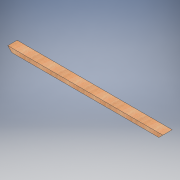
# Autodesk Inventor part: 58 Inch 45 Diagonal Piece
Saved by Autodesk Inventor 2016 (Build 200138000, 138)
## iProperties
Created: 2015-07-05
Part Number: 58 Inch 45 Diagonal Piece
Material: Wood (Birch)
Document SubType Name: Modeling
Designer: steele
Density: 0.55 g/cm^3
Appearance: Birch - Natural Polished
Author: steele
Autodesk Inventor part; units mm, degrees
ref_plane "YZ Plane" through (0, 0, 0) normal (1, 0, 0) x (0, 1, 0)
ref_plane "XZ Plane" through (0, 0, 0) normal (0, 1, 0) x (-1, 0, 0)
ref_plane "XY Plane" through (0, 0, 0) normal (0, 0, 1) x (1, 0, 0)
sketch "Sketch2" plane through (0, 0, 0) normal (0, 0, 1) x (1, 0, 0)
  line L0 (-698.5, -19.05) -> (698.5, -19.05)
  line L1 (736.6, 19.05) -> (-736.6, 19.05)
  line L2 (-736.6, -19.05) -> (736.6, 19.05) construction
  line L3 (736.6, -19.05) -> (-736.6, 19.05) construction
  line L4 (-736.6, 19.05) -> (-698.5, -19.05)
  line L5 (-736.6, 19.05) -> (-682.7185, 19.05) construction
  line L6 (736.6, 19.05) -> (698.5, -19.05)
  line L7 (736.6, 19.05) -> (790.4815, 19.05) construction
  point P0 (0, 0)
  dimension "d10" = 45
  dimension "d11" = 135
  dimension "d14" = 1473.2
  dimension "d15" = 38.1
  constraints: 16 end point, 3 horizontal, 2 equal length, 2 midpoint, 1 parallel
  measures "d10" angle of L4 L5
  measures "d11" angle of L6 L7
  measures "d14" distance of L1.start L1.end
  measures "d15" distance between parallel lines of L0 L1
extrude "Extrusion2" add sketch "Sketch2" along normal mid plane 88.9
body "Solid2"
